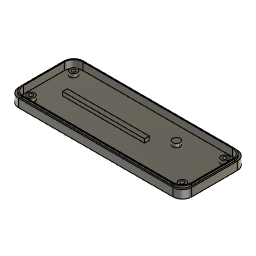
Macropad_V1_Case (Autodesk Fusion 360 design; units mm, degrees)
Autodesk Fusion 360 part; units mm, degrees
sketch "PCB" plane through (0, 0, 0) normal (0, 0, 1) x (1, 0, 0)
  line L0 (0, 0) -> (129.54, 0)
  line L1 (129.54, 0) -> (129.54, 41.91)
  line L2 (129.54, 41.91) -> (0, 41.91)
  line L3 (0, 41.91) -> (0, 0)
  circle A0 centre (3.81, 38.1) radius 1
  circle A1 centre (3.81, 3.81) radius 1
  circle A2 centre (125.73, 3.81) radius 1
  circle A3 centre (125.73, 38.1) radius 1
  line L4 (7.62, 38.1) -> (22.86, 38.1)
  line L5 (22.86, 38.1) -> (22.86, 22.86)
  line L6 (22.86, 22.86) -> (7.62, 22.86)
  line L7 (7.62, 22.86) -> (7.62, 38.1)
  line L8 (26.67, 22.86) -> (26.67, 38.1)
  line L9 (26.67, 38.1) -> (41.91, 38.1)
  line L10 (41.91, 38.1) -> (41.91, 22.86)
  line L11 (41.91, 22.86) -> (26.67, 22.86)
  line L12 (45.72, 22.86) -> (45.72, 38.1)
  line L13 (45.72, 38.1) -> (60.96, 38.1)
  line L14 (60.96, 38.1) -> (60.96, 22.86)
  line L15 (60.96, 22.86) -> (45.72, 22.86)
  line L16 (64.77, 22.86) -> (64.77, 38.1)
  line L17 (64.77, 38.1) -> (80.01, 38.1)
  line L18 (80.01, 38.1) -> (80.01, 22.86)
  line L19 (80.01, 22.86) -> (64.77, 22.86)
  line L20 (13.97, 19.05) -> (29.21, 19.05)
  line L21 (29.21, 19.05) -> (29.21, 3.81)
  line L22 (29.21, 3.81) -> (13.97, 3.81)
  line L23 (13.97, 3.81) -> (13.97, 19.05)
  line L24 (33.02, 3.81) -> (33.02, 19.05)
  line L25 (33.02, 19.05) -> (48.26, 19.05)
  line L26 (48.26, 19.05) -> (48.26, 3.81)
  line L27 (48.26, 3.81) -> (33.02, 3.81)
  line L28 (52.07, 3.81) -> (52.07, 19.05)
  line L29 (52.07, 19.05) -> (67.31, 19.05)
  line L30 (67.31, 19.05) -> (67.31, 3.81)
  line L31 (67.31, 3.81) -> (52.07, 3.81)
  line L32 (71.12, 3.81) -> (71.12, 19.05)
  line L33 (71.12, 19.05) -> (86.36, 19.05)
  line L34 (86.36, 19.05) -> (86.36, 3.81)
  line L35 (86.36, 3.81) -> (71.12, 3.81)
  line L36 (104.14, 41.91) -> (121.92, 41.91)
  line L37 (121.92, 41.91) -> (121.92, 8.89)
  line L38 (121.92, 8.89) -> (104.14, 8.89)
  line L39 (104.14, 8.89) -> (104.14, 41.91)
  line L40 (115.65, 6.27) -> (120.65, 6.27)
  line L41 (120.65, 6.27) -> (120.65, 1.27)
  line L42 (120.65, 1.27) -> (115.65, 1.27)
  line L43 (115.65, 1.27) -> (115.65, 6.27)
  line L44 (104.22, 1.27) -> (104.22, 6.27)
  line L45 (104.22, 6.27) -> (109.22, 6.27)
  line L46 (109.22, 6.27) -> (109.22, 1.27)
  line L47 (109.22, 1.27) -> (104.22, 1.27)
  line L48 (92.79, 1.27) -> (92.79, 6.27)
  line L49 (92.79, 6.27) -> (97.79, 6.27)
  line L50 (97.79, 6.27) -> (97.79, 1.27)
  line L51 (97.79, 1.27) -> (92.79, 1.27)
  circle A4 centre (93.98, 30.734) radius 3.81
  dimension "d1" = 129.54
  dimension "d2" = 41.91
  dimension "d38" = 2
  dimension "d39" = 3.81
  dimension "d40" = 3.81
  dimension "d41" = 2
  dimension "d42" = 3.81
  dimension "d43" = 3.81
  dimension "d44" = 2
  dimension "d45" = 3.81
  dimension "d46" = 3.81
  dimension "d47" = 2
  dimension "d48" = 3.81
  dimension "d49" = 3.81
  dimension "d50" = 15.24
  dimension "d51" = 15.24
  dimension "d52" = 7.62
  dimension "d53" = 3.81
  dimension "d56" = 19.05
  dimension "d57" = 0
  dimension "d58" = 15.24
  dimension "d59" = 15.24
  dimension "d60" = 19.05
  dimension "d61" = 6.35
  dimension "d64" = 19.05
  dimension "d65" = 0
  dimension "d66" = 17.78
  dimension "d67" = 33.02
  dimension "d68" = 7.62
  dimension "d71" = 5
  dimension "d72" = 5
  dimension "d73" = 8.89
  dimension "d74" = 1.27
  dimension "d77" = -11.43
  dimension "d78" = 0
  dimension "d79" = 7.62
  dimension "d80" = 35.56
  dimension "d81" = 11.176
  constraint horizontal L0
  constraint vertical L1
  constraint horizontal L2
  constraint vertical L3
  constraint coincident L0.start L3.end
  constraint horizontal L4
  constraint vertical L5
  constraint horizontal L6
  constraint vertical L7
  constraint horizontal L20
  constraint vertical L21
  constraint horizontal L22
  constraint vertical L23
  constraint horizontal L36
  constraint vertical L37
  constraint horizontal L38
  constraint vertical L39
  constraint collinear L2 L36
  constraint horizontal L40
  constraint vertical L41
  constraint horizontal L42
  constraint vertical L43
  measures "d1" distance of L0.start L0.end
  measures "d2" distance of L0.start L2.end
  measures "d38" diameter of A0
  measures "d39" distance of L3 A0.centre
  measures "d40" distance of L2 A0.centre
  measures "d41" diameter of A1
  measures "d42" distance of L0 A1.centre
  measures "d43" distance of L3 A1.centre
  measures "d44" diameter of A2
  measures "d45" distance of L1 A2.centre
  measures "d46" distance of L0 A2.centre
  measures "d47" diameter of A3
  measures "d48" distance of L2 A3.centre
  measures "d49" distance of L1 A3.centre
  measures "d50" distance of L4.start L4.end
  measures "d51" distance of L4.start L6.end
  measures "d52" distance of L3 L7
  measures "d53" distance of L2 L4
  measures "d58" distance of L20.end L20.start
  measures "d59" distance of L22.end L20.start
  measures "d60" distance of L4 L20
  measures "d61" distance of L7 L23
  measures "d66" distance of L36.start L36.end
  measures "d67" distance of L36.start L38.end
  measures "d68" distance of L1 L37
  measures "d71" distance of L40.start L40.end
  measures "d72" distance of L40.start L42.end
  measures "d73" distance of L1 L41
  measures "d74" distance of L0 L42
  measures "d79" diameter of A4
  measures "d80" distance of L1 A4.centre
  measures "d81" distance of L2 A4.centre
sketch "Bottom" plane through (0, 0, 0) normal (0, 0, 1) x (1, 0, 0)
  line L0 (2.5, 46.91) -> (127.04, 46.91)
  line L1 (134.54, 39.41) -> (134.54, 2.5)
  line L2 (127.04, -5) -> (2.5, -5)
  line L3 (-5, 2.5) -> (-5, 39.41)
  line L4 (0, 41.91) -> (0, 0)
  line L5 (129.54, 0) -> (129.54, 41.91)
  line L6 (129.54, 41.91) -> (0, 41.91)
  line L7 (0, 0) -> (129.54, 0)
  arc A0 (2.5, 46.91) -> (-5, 39.41) centre (2.5, 39.41) ccw
  arc A1 (134.54, 39.41) -> (127.04, 46.91) centre (127.04, 39.41) ccw
  arc A2 (127.04, -5) -> (134.54, 2.5) centre (127.04, 2.5) ccw
  arc A3 (-5, 2.5) -> (2.5, -5) centre (2.5, 2.5) ccw
  dimension "d9" = 5
  dimension "d10" = 5
  dimension "d11" = 5
  dimension "d12" = 5
  dimension "d13" = 7.5
  constraint horizontal L0
  constraint vertical L1
  constraint horizontal L2
  constraint vertical L3
  constraint tangent L3 A0
  constraint tangent L0 A0
  constraint tangent L0 A1
  constraint tangent L1 A1
  constraint equal A0 A1
  constraint tangent L1 A2
  constraint tangent L2 A2
  constraint equal A0 A2
  constraint tangent L2 A3
  constraint tangent L3 A3
  constraint equal A0 A3
  measures "d9" distance of L3 L4
  measures "d10" distance of L1 L5
  measures "d11" distance of L0 L6
  measures "d12" distance of L2 L7
  measures "d13" radius of A0
extrude "Extrude1" add sketch "Bottom" along normal blind 6.6 contours L0 L1 L2 L3 A0 A1 A2 A3 | L4 L5 L6 L7
sketch "Bottom indent" plane through (0, 0, 6.6) normal (0, 0, 1) x (-1, 0, 0)
  arc A0 (-2.5, -46.91) -> (5, -39.41) centre (-2.5, -39.41) ccw
  line L0 (5, -39.41) -> (5, -2.5)
  arc A1 (5, -2.5) -> (-2.5, 5) centre (-2.5, -2.5) ccw
  line L1 (-2.5, 5) -> (-127.04, 5)
  arc A2 (-127.04, 5) -> (-134.54, -2.5) centre (-127.04, -2.5) ccw
  line L2 (-134.54, -2.5) -> (-134.54, -39.41)
  arc A3 (-134.54, -39.41) -> (-127.04, -46.91) centre (-127.04, -39.41) ccw
  line L3 (-127.04, -46.91) -> (-2.5, -46.91)
  line L4 (-4.5, -44.91) -> (-125.04, -44.91)
  line L5 (-132.54, -37.41) -> (-132.54, -4.5)
  line L6 (-125.04, 3) -> (-4.5, 3)
  line L7 (3, -4.5) -> (3, -37.41)
  arc A4 (-4.5, -44.91) -> (3, -37.41) centre (-4.5, -37.41) ccw
  arc A5 (-132.54, -37.41) -> (-125.04, -44.91) centre (-125.04, -37.41) ccw
  arc A6 (-125.04, 3) -> (-132.54, -4.5) centre (-125.04, -4.5) ccw
  arc A7 (3, -4.5) -> (-4.5, 3) centre (-4.5, -4.5) ccw
  dimension "d17" = 2
  dimension "d18" = 2
  dimension "d19" = 2
  dimension "d20" = 2
  dimension "d21" = 7.5
  constraint horizontal L4
  constraint vertical L5
  constraint horizontal L6
  constraint vertical L7
  constraint tangent L7 A4
  constraint tangent L4 A4
  constraint tangent L4 A5
  constraint tangent L5 A5
  constraint equal A4 A5
  constraint tangent L5 A6
  constraint tangent L6 A6
  constraint equal A4 A6
  constraint tangent L6 A7
  constraint tangent L7 A7
  constraint equal A4 A7
  measures "d17" distance of L0 L7
  measures "d18" distance of L2 L5
  measures "d19" distance of L3 L4
  measures "d20" distance of L1 L6
  measures "d21" radius of A4
extrude "Extrude2" cut sketch "Bottom indent" against normal blind 4.6 contours L4 L5 L6 L7 A4 A5 A6 A7
sketch "Feet holes" plane through (0, 0, 0) normal (0, 0, -1) x (1, 0, 0)
  arc A0 (-5, -39.41) -> (2.5, -46.91) centre (2.5, -39.41) ccw
  line L0 (2.5, -46.91) -> (127.04, -46.91)
  arc A1 (127.04, -46.91) -> (134.54, -39.41) centre (127.04, -39.41) ccw
  line L1 (134.54, -39.41) -> (134.54, -2.5)
  arc A2 (134.54, -2.5) -> (127.04, 5) centre (127.04, -2.5) ccw
  line L2 (127.04, 5) -> (2.5, 5)
  arc A3 (2.5, 5) -> (-5, -2.5) centre (2.5, -2.5) ccw
  line L3 (-5, -2.5) -> (-5, -39.41)
  circle A4 centre (5, -5) radius 5
  circle A5 centre (5, -36.91) radius 5
  circle A6 centre (124.54, -5) radius 5
  circle A7 centre (124.54, -36.91) radius 5
  dimension "d24" = 10
  dimension "d25" = 10
  dimension "d26" = 10
  dimension "d27" = 10
  dimension "d28" = 10
  dimension "d29" = 10
  dimension "d30" = 10
  dimension "d31" = 10
  dimension "d32" = 10
  dimension "d33" = 10
  dimension "d34" = 10
  dimension "d35" = 10
  measures "d24" diameter of A4
  measures "d25" distance of L2 A4.centre
  measures "d26" distance of L3 A4.centre
  measures "d27" diameter of A5
  measures "d28" diameter of A6
  measures "d29" diameter of A7
  measures "d30" distance of L3 A5.centre
  measures "d31" distance of L0 A5.centre
  measures "d32" distance of L1 A6.centre
  measures "d33" distance of L2 A6.centre
  measures "d34" distance of L1 A7.centre
  measures "d35" distance of L0 A7.centre
extrude "Extrude3" cut sketch "Feet holes" against normal blind 1 contours A4 | A5 | A6 | A7
sketch "Bottom risers" plane through (0, 0, 2) normal (0, 0, 1) x (-1, 0, 0)
  arc A0 (-4.5, -44.91) -> (3, -37.41) centre (-4.5, -37.41) ccw
  line L0 (3, -37.41) -> (3, -4.5)
  arc A1 (3, -4.5) -> (-4.5, 3) centre (-4.5, -4.5) ccw
  line L1 (-4.5, 3) -> (-125.04, 3)
  arc A2 (-125.04, 3) -> (-132.54, -4.5) centre (-125.04, -4.5) ccw
  line L2 (-132.54, -4.5) -> (-132.54, -37.41)
  arc A3 (-132.54, -37.41) -> (-125.04, -44.91) centre (-125.04, -37.41) ccw
  line L3 (-125.04, -44.91) -> (-4.5, -44.91)
  circle A4 centre (-3.81, -38.1) radius 3
  circle A5 centre (-3.81, -38.1) radius 1
  circle A6 centre (-3.81, -3.81) radius 3
  circle A7 centre (-125.73, -38.1) radius 3
  circle A8 centre (-125.73, -3.81) radius 3
  circle A9 centre (-3.81, -3.81) radius 1
  circle A10 centre (-125.73, -38.1) radius 1
  circle A11 centre (-125.73, -3.81) radius 1
  line L4 (-13.97, -22.86) -> (-80.01, -22.86)
  line L5 (-80.01, -22.86) -> (-80.01, -19.05)
  line L6 (-80.01, -19.05) -> (-13.97, -19.05)
  line L7 (-13.97, -19.05) -> (-13.97, -22.86)
  line L8 (-80.01, -38.1) -> (-80.01, -22.86)
  line L9 (-13.97, -3.81) -> (-13.97, -19.05)
  line L10 (-13.97, -19.05) -> (-29.21, -19.05)
  line L11 (-80.01, -22.86) -> (-64.77, -22.86)
  circle A12 centre (-93.98, -30.734) radius 3
  circle A13 centre (-93.98, -30.734) radius 3.81
  circle A14 centre (-3.81, -38.1) radius 1.5
  circle A15 centre (-3.81, -3.81) radius 1.5
  circle A16 centre (-125.73, -3.81) radius 1.5
  circle A17 centre (-125.73, -38.1) radius 1.5
  dimension "d82" = 6
  dimension "d83" = 6
  dimension "d84" = 6
  dimension "d85" = 6
  dimension "d87" = 6
  dimension "d88" = 3
  dimension "d89" = 3
  dimension "d90" = 3
  dimension "d91" = 3
  constraint concentric A4 A5
  constraint concentric A6 A9
  constraint concentric A7 A10
  constraint concentric A8 A11
  constraint horizontal L4
  constraint vertical L5
  constraint horizontal L6
  constraint vertical L7
  constraint collinear L5 L8
  constraint collinear L7 L9
  constraint collinear L6 L10
  constraint collinear L4 L11
  constraint concentric A12 A13
  constraint concentric A5 A14
  constraint concentric A9 A15
  constraint concentric A11 A16
  constraint concentric A10 A17
  measures "d82" diameter of A4
  measures "d83" diameter of A6
  measures "d84" diameter of A7
  measures "d85" diameter of A8
  measures "d87" diameter of A12
  measures "d88" diameter of A14
  measures "d89" diameter of A15
  measures "d90" diameter of A16
  measures "d91" diameter of A17
extrude "Extrude4" add sketch "Bottom risers" along normal blind 3 contours A4 | A6 | A7 | A8 | L4 L5 L6 L7 L10 L11 | A12
extrude "Extrude5" cut 4 faces at (4.4705, 37.7379, 2) (3.6858, 4.5903, 2) (125.6187, 38.5875, 2) (126.2643, 4.2009, 2) along direction (0, 0, -1) blind 1
sketch "Bottom Raised Edge" plane through (0, 0, 6.6) normal (0, 0, 1) x (-1, 0, 0)
  line L0 (3, -4.5) -> (3, -37.41)
  arc A0 (-4.5, -44.91) -> (3, -37.41) centre (-4.5, -37.41) ccw
  line L1 (-4.5, -44.91) -> (-125.04, -44.91)
  arc A1 (-132.54, -37.41) -> (-125.04, -44.91) centre (-125.04, -37.41) ccw
  line L2 (-132.54, -37.41) -> (-132.54, -4.5)
  arc A2 (-125.04, 3) -> (-132.54, -4.5) centre (-125.04, -4.5) ccw
  line L3 (-125.04, 3) -> (-4.5, 3)
  arc A3 (3, -4.5) -> (-4.5, 3) centre (-4.5, -4.5) ccw
  arc A4 (-2.5, -46.91) -> (5, -39.41) centre (-2.5, -39.41) ccw
  line L4 (5, -39.41) -> (5, -2.5)
  arc A5 (5, -2.5) -> (-2.5, 5) centre (-2.5, -2.5) ccw
  line L5 (-2.5, 5) -> (-127.04, 5)
  arc A6 (-127.04, 5) -> (-134.54, -2.5) centre (-127.04, -2.5) ccw
  line L6 (-134.54, -2.5) -> (-134.54, -39.41)
  arc A7 (-134.54, -39.41) -> (-127.04, -46.91) centre (-127.04, -39.41) ccw
  line L7 (-127.04, -46.91) -> (-2.5, -46.91)
  line L8 (-3.7, -45.71) -> (-125.84, -45.71)
  line L9 (-133.34, -38.21) -> (-133.34, -3.7)
  line L10 (-125.84, 3.8) -> (-3.7, 3.8)
  line L11 (3.8, -3.7) -> (3.8, -38.21)
  arc A8 (-3.7, -45.71) -> (3.8, -38.21) centre (-3.7, -38.21) ccw
  arc A9 (-133.34, -38.21) -> (-125.84, -45.71) centre (-125.84, -38.21) ccw
  arc A10 (-125.84, 3.8) -> (-133.34, -3.7) centre (-125.84, -3.7) ccw
  arc A11 (3.8, -3.7) -> (-3.7, 3.8) centre (-3.7, -3.7) ccw
  dimension "d96" = 0.8
  dimension "d97" = 0.8
  dimension "d98" = 0.8
  dimension "d100" = 0.8
  dimension "d101" = 7.5
  constraint horizontal L8
  constraint vertical L9
  constraint horizontal L10
  constraint vertical L11
  constraint tangent L8 A8
  constraint tangent L11 A8
  constraint tangent L8 A9
  constraint tangent L9 A9
  constraint equal A8 A9
  constraint tangent L9 A10
  constraint tangent L10 A10
  constraint equal A8 A10
  constraint tangent L10 A11
  constraint tangent L11 A11
  constraint equal A8 A11
  measures "d96" distance of L1 L8
  measures "d97" distance of L0 L11
  measures "d98" distance of L2 L9
  measures "d100" distance of L3 L10
  measures "d101" radius of A8
extrude "Extrude6" add sketch "Bottom Raised Edge" along normal blind 1.4 contours L8 L9 L10 L11 A8 A9 A10 A11
equation "d14 = 2 mm + 3 mm + 1.6 mm"
equation "d22 = -3 mm - 1.6 mm"
equation "d77 = ( -4.5 * 2.54 ) * 1 mm"
named bodies: "Bottom"
